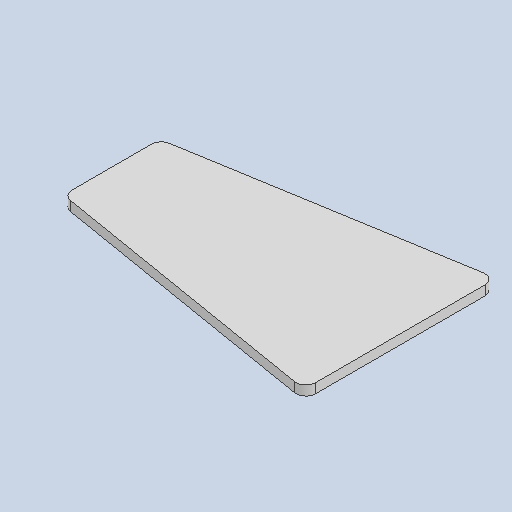
# Autodesk Inventor part: Stand
Saved by Autodesk Inventor 2022 (Build 260153000, 153)
## iProperties
Created: 2020-11-05
Part Number: Stand
Material: Generic
Document SubType Name: Modeling
Designer: simen
Density: 1 g/cm^3
Appearance: Default
Author: simen
Autodesk Inventor part; units mm, degrees
ref_plane "YZ Plane" through (0, 0, 0) normal (1, 0, 0) x (0, 1, 0)
ref_plane "XZ Plane" through (0, 0, 0) normal (0, 1, 0) x (-1, 0, 0)
ref_plane "XY Plane" through (0, 0, 0) normal (0, 0, 1) x (1, 0, 0)
sketch "Sketch1" plane through (0, 0, 0) normal (0, 1, 0) x (-1, 0, 0)
  line L0 (42.3662, 9.0765) -> (-13.6338, 18.4098)
  line L1 (-15.9626, 16.437) -> (-15.9626, -18.8411)
  line L2 (-13.6338, -20.8139) -> (42.3662, -11.4806)
  line L3 (44.0374, -9.5078) -> (44.0374, 7.1037)
  line L4 (44.0374, -1.202) -> (-15.9626, -1.202) construction
  arc A0 (-13.6338, 18.4098) -> (-15.9626, 16.437) centre (-13.9626, 16.437) ccw
  arc A1 (-15.9626, -18.8411) -> (-13.6338, -20.8139) centre (-13.9626, -18.8411) ccw
  arc A2 (44.0374, 7.1037) -> (42.3662, 9.0765) centre (42.0374, 7.1037) ccw
  arc A3 (42.3662, -11.4806) -> (44.0374, -9.5078) centre (42.0374, -9.5078) ccw
  point P0 (0, 0)
  point P1 (44.0374, 8.798)
  point P2 (-15.9626, -21.202)
  point P3 (-15.9626, 18.798)
  point P4 (44.0374, -11.202)
  dimension "d4" = 40
  dimension "d5" = 20
  dimension "d6" = 60
  dimension "d7" = 2
  constraints: 10 end point, 8 point on circle, 8 point on line, 8 tangent, 4 centre point, 3 equal radius, 2 midpoint, 1 parallel, 1 perpendicular, 1 vertical
  measures "d4" distance of point (-15.963, 18.798) point (-15.963, -21.202)
  measures "d5" distance of point (44.037, -11.202) point (44.037, 8.798)
  measures "d6" distance of L4.start L4.end
  measures "d7" radius of A0
extrude "Extrusion1" add sketch "Sketch1" along normal blind 2
body "Solid1"
